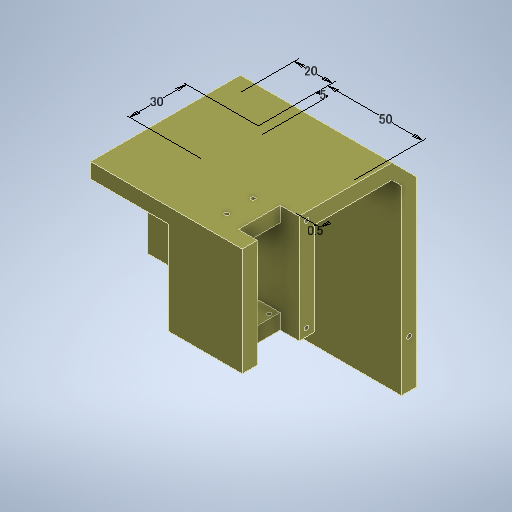
# Autodesk Inventor part: 左仕切り
Saved by Autodesk Inventor 2026.2 (Build 302298010, 298A)
## iProperties
Created: 2026-05-20
Part Number: 左仕切り
Material: 一般
Document SubType Name: Modeling
Designer: Yagis
Density: 1 g/cm^3
Appearance: 既定
Mass: 220.852 g
Surface Area: 622.361 cm^2
Volume: 220.852 cm^3
Author: Yagis
Autodesk Inventor part; units mm, degrees
ref_plane "YZ Plane" through (0, 0, 0) normal (1, 0, 0) x (0, 1, 0)
ref_plane "XZ Plane" through (0, 0, 0) normal (0, 1, 0) x (-1, 0, 0)
ref_plane "XY Plane" through (0, 0, 0) normal (0, 0, 1) x (1, 0, 0)
sketch "スケッチ1" plane through (0, 0, 0) normal (1, 0, 0) x (0, 1, 0)
  line L0 (0, 0) -> (-96, 0)
  line L1 (-96, 0) -> (-96, -8)
  line L2 (-96, -8) -> (0, -8)
  line L3 (0, -8) -> (0, 0)
  line L4 (13, 5) -> (5, 5)
  line L5 (5, 5) -> (5, 75)
  line L6 (5, 75) -> (13, 75)
  line L7 (13, 75) -> (13, 5)
  line L8 (13, 5) -> (0, -8)
  line L9 (5, 5) -> (0, 0)
  line L10 (-44, 84) -> (13, 84)
  line L11 (13, 84) -> (13, 75)
  line L12 (-44, 76) -> (-44, 46)
  line L13 (-44, 46) -> (-36, 46)
  line L14 (-36, 46) -> (-36, 76)
  line L15 (5, 75) -> (5, 76)
  line L16 (5, 76) -> (-44, 76)
  line L17 (-44, 84) -> (-44, 76)
  point P0 (-36, 0)
  point P1 (-36, 76)
  point P2 (-44, 76)
  dimension "d11" = 6
  dimension "d0" = 8
  dimension "d2" = 8
  dimension "d3" = 70
  dimension "d4" = 96
  dimension "d17" = 13
  dimension "d36" = 8
  dimension "d37" = 41
  dimension "d53" = 1
  dimension "d54" = 8
  dimension "d55" = 30
  dimension "d72" = 57
  dimension "d86" = 30
  constraints: 36 end point, 5 parallel, 4 perpendicular, 2 horizontal, 2 vertical, 1 point on line
  measures "d0" distance of L0.end L1.end
  measures "d2" distance between parallel lines of L5 L7
  measures "d3" distance of L4.end L5.end
  measures "d4" distance of L0.start L0.end
  measures "d17" distance from line of L2.end L4
  measures "d36" distance between parallel lines of L12 L14
  measures "d37" distance between parallel lines of L14 L5
  measures "d53" distance of L5.end L15.end
  measures "d54" distance between parallel lines of L10 L16
  measures "d55" distance of L13.end L14.end
  measures "d72" distance between parallel lines of L17 L11
  measures "d86" distance of L12.start L12.end
extrude "押し出し1" add sketch "スケッチ1" along normal blind 80
sketch "スケッチ2" plane through (80, 0, 0) normal (1, 0, 0) x (0, 0, -1)
  line L0 (8, -96) -> (8, 0) projected
  point P0 (0, 0)
  point P1 (4, -71)
  point P2 (-50, 9)
  point P3 (-50, -40)
  dimension "d9" = 4
  dimension "d19" = 80
  dimension "d84" = 58
  dimension "d87" = 49
  constraints: 1 vertical alignment
  measures "d9" distance from line of L0 point (4, -71)
  measures "d19" vertical distance of point (4, -71) point (-50, 9)
  measures "d84" distance from line of L0 point (-50, 9)
  measures "d87" distance of point (-50, -40) point (-50, 9)
hole "穴1" at (80, -71, -4) at (80, 9, 50) at (80, -40, 50) direction (-1, 0, 0) diameter 2.459 depth 8.8 tip angle 118 thread size "M3x0.5" class "6H" standard "ISO Metric profile"
sketch "スケッチ5" plane through (0, 13, 84) normal (0, 1, 0) x (1, 0, 0)
  line L0 (80, 8) -> (70, 8)
  line L1 (70, 8) -> (70, 30)
  line L2 (70, 30) -> (80, 30)
  line L3 (80, 30) -> (80, 8)
  line L4 (0, 0) -> (80, 0) projected
  line L5 (80, 79) -> (80, 0) projected
  point P0 (0, 84)
  dimension "d38" = 8
  dimension "d39" = 10
  dimension "d40" = 22
  constraints: 8 end point, 2 parallel, 1 collinear, 1 horizontal, 1 perpendicular
  measures "d38" distance between parallel lines of L0 L4
  measures "d39" distance between parallel lines of L1 L3
  measures "d40" distance between parallel lines of L0 L2
extrude "押し出し3" cut sketch "スケッチ5" against normal blind 80
sketch "スケッチ6" plane through (0, 13, 84) normal (0, 1, 0) x (1, 0, 0)
  line L0 (80, 8) -> (80, 0) projected
  line L1 (0, 0) -> (80, 0) projected
  point P0 (0, 84)
  point P1 (59.78, 12)
  point P2 (59.78, 26)
  dimension "d43" = 20.22
  dimension "d44" = 12
  dimension "d45" = 14
  constraints: 1 vertical alignment
  measures "d43" distance from line of point (59.78, 12) L0
  measures "d44" distance from line of L1 point (59.78, 12)
  measures "d45" distance of point (59.78, 26) point (59.78, 12)
hole "穴3" at (59.78, 13, 72) at (59.78, 13, 58) direction (0, -1, 0) diameter 2.2 depth 8.8 tip angle 118
sketch "スケッチ7" plane through (0, -44, 46) normal (0, -1, 0) x (1, 0, 0)
  line L0 (80, 8) -> (80, 0) projected
  line L1 (80, 8) -> (70, 8) projected
  point P0 (0, -46)
  point P1 (67.7, 26.5)
  point P2 (67.7, 11.5)
  point P3 (52.7, 26.5)
  point P4 (52.7, 11.5)
  dimension "d58" = 15
  dimension "d59" = 15
  dimension "d60" = 12.3
  dimension "d61" = 3.5
  constraints: 2 horizontal alignment, 2 vertical alignment
  measures "d58" distance of point (67.7, 26.5) point (67.7, 11.5)
  measures "d59" distance of point (52.7, 26.5) point (67.7, 26.5)
  measures "d60" distance from line of point (67.7, 11.5) L0
  measures "d61" distance from line of L1 point (67.7, 11.5)
hole "穴4" at (67.7, -44, 72.5) at (67.7, -44, 57.5) at (52.7, -44, 72.5) at (52.7, -44, 57.5) direction (0, 1, 0) diameter 2.2 depth 8 tip angle 118
sketch "スケッチ8" plane through (0, -44, 46) normal (0, -1, 0) x (1, 0, 0)
  line L0 (0, 38) -> (41.2, 38)
  line L1 (41.2, 38) -> (41.2, 8)
  line L2 (41.2, 8) -> (0, 8)
  line L3 (0, 8) -> (0, 38)
  line L4 (0, -46) -> (80, -46) projected
  line L5 (0, 38) -> (0, -46) projected
  line L6 (0, 38) -> (80, 38) projected
  circle A0 centre (52.7, 26.5) radius 1.1 projected
  line L7 (80, 8) -> (70, 8) projected
  dimension "d75" = 11.5
  dimension "d83" = 0
  constraints: 8 end point, 2 collinear, 2 parallel, 1 horizontal, 1 perpendicular, 1 other
  measures "d75" distance from line of L1 A0.centre
  measures "d83" distance between parallel lines of L7 L2
extrude "押し出し4" cut sketch "スケッチ8" against normal blind 10 contours L0 L1 L2 L3
sketch "スケッチ9" plane through (0, -34, 46) normal (0, -1, 0) x (1, 0, 0)
  point P0 (0, -46)
sketch "スケッチ10" plane through (0, -34, 46) normal (0, -1, 0) x (1, 0, 0)
  line L0 (41.2, 38) -> (0, 38)
  line L1 (0, 38) -> (0, 30)
  line L2 (0, 30) -> (41.2, 30)
  line L3 (41.2, 30) -> (41.2, 38)
  line L4 (0, 38) -> (41.2, 38) projected
  line L5 (41.2, 38) -> (41.2, 8) projected
  line L6 (0, 30) -> (0, 38) projected
  line L7 (41.2, 30) -> (0, 30) projected
  point P0 (0, -46)
  point P1 (41.2, 0)
  constraints: 8 end point, 4 collinear, 2 parallel, 1 horizontal, 1 perpendicular
extrude "押し出し5" cut sketch "スケッチ10" against normal blind 39
sketch "スケッチ11" plane through (0, 5, 5) normal (0, -1, 0) x (1, 0, 0)
  point P0 (0, -5)
sketch "スケッチ12" plane through (0, 5, 5) normal (0, -1, 0) x (1, 0, 0)
  line L0 (41.2, 71) -> (49.2, 71)
  line L1 (49.2, 71) -> (49.2, 49)
  line L2 (49.2, 49) -> (41.2, 49)
  line L3 (41.2, 49) -> (41.2, 71)
  point P0 (0, -5)
  point P1 (70, 71)
  point P2 (41.2, 71)
  dimension "d76" = 8
  dimension "d77" = 22
  constraints: 8 end point, 2 parallel, 1 coincident, 1 horizontal, 1 horizontal alignment, 1 perpendicular
  measures "d76" distance between parallel lines of L1 L3
  measures "d77" distance of L0.end L1.end
extrude "押し出し6" add sketch "スケッチ12" along normal blind 49
sketch "スケッチ13" plane through (80, 0, 0) normal (1, 0, 0) x (0, 0, -1)
  line L0 (-54, 5) -> (-46, 5)
  line L1 (-46, 5) -> (-46, -36)
  line L2 (-46, -36) -> (-54, -36)
  line L3 (-54, -36) -> (-54, 5)
  line L4 (-54, 5) -> (-5, 5) projected
  line L5 (-46, -36) -> (-54, -36) projected
  line L6 (-54, 5) -> (-54, -36) projected
  line L7 (-46, -44) -> (-46, -36) projected
  point P0 (0, 0)
  constraints: 8 end point, 4 collinear, 2 parallel, 1 horizontal, 1 perpendicular
extrude "押し出し7" add sketch "スケッチ13" against normal blind 80
sketch "スケッチ14" plane through (0, 5, 46) normal (0, -1, 0) x (1, 0, 0)
  line L0 (70, -0.5) -> (20, -0.5)
  line L1 (20, -0.5) -> (20, -30.5)
  line L2 (20, -30.5) -> (70, -30.5)
  line L3 (70, -30.5) -> (70, -0.5)
  line L4 (0, -41) -> (0, 0) projected
  line L5 (0, 0) -> (80, 0) projected
  line L6 (66.594, -2.5303) -> (25, -2.5303)
  line L7 (25, -2.5303) -> (25, -27.2887)
  line L8 (25, -27.2887) -> (66.594, -27.2887)
  line L9 (66.594, -27.2887) -> (66.594, -2.5303)
  point P0 (0, -46)
  point P1 (0, -20.5)
  dimension "d88" = 20
  dimension "d89" = 30
  dimension "d90" = 50
  dimension "d91" = 0.5
  dimension "d92" = 5
  constraints: 16 end point, 4 parallel, 2 horizontal, 2 perpendicular, 1 midpoint
  measures "d88" distance between parallel lines of L4 L1
  measures "d89" distance between parallel lines of L2 L0
  measures "d90" distance of L1.end L2.end
  measures "d91" distance between parallel lines of L5 L0
  measures "d92" distance between parallel lines of L7 L1
